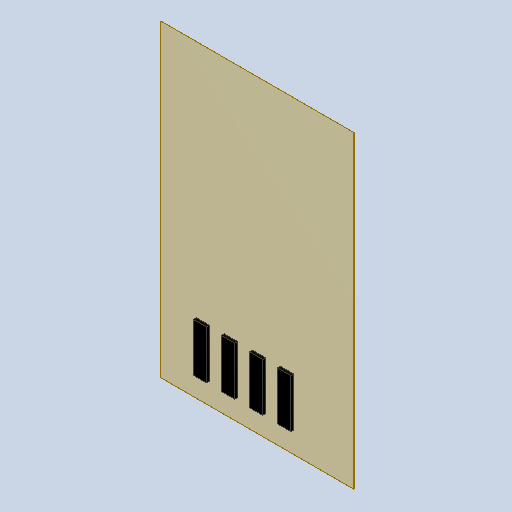
# Autodesk Inventor part: dirt
Saved by Autodesk Inventor 2025 (Build 290162010, 162A)
## iProperties
Created: 2024-06-18
Part Number: dirt
Material: 일반
Document SubType Name: Modeling
Designer: user
Density: 1 g/cm^3
Appearance: 기본값
Author: user
Autodesk Inventor part; units mm, degrees
ref_plane "YZ Plane" through (0, 0, 0) normal (1, 0, 0) x (0, 1, 0)
ref_plane "XZ Plane" through (0, 0, 0) normal (0, 1, 0) x (-1, 0, 0)
ref_plane "XY Plane" through (0, 0, 0) normal (0, 0, 1) x (1, 0, 0)
ref_plane "작업 평면1" through (2977.2317, -10029.2607, -15) normal (0, 0, 1) x (1, 0, 0)
ref_plane "작업 평면2" through (2977.2317, -10029.2607, -30) normal (0, 0, 1) x (1, 0, 0)
sketch "스케치1" plane through (2977.2317, -10029.2607, -30) normal (0, 0, 1) x (1, 0, 0)
  line L0 (5170.4623, -12069.2506) -> (3270.4623, -12069.2506)
  line L1 (3270.4623, -12069.2506) -> (3270.4623, -18969.2506)
  line L2 (3270.4623, -18969.2506) -> (5170.4623, -18969.2506)
  line L3 (5170.4623, -18969.2506) -> (5170.4623, -12069.2506)
  line L4 (1170.4623, -12069.2506) -> (-729.5377, -12069.2506)
  line L5 (-729.5377, -12069.2506) -> (-729.5377, -18969.2506)
  line L6 (-729.5377, -18969.2506) -> (1170.4623, -18969.2506)
  line L7 (1170.4623, -18969.2506) -> (1170.4623, -12069.2506)
  line L8 (-2829.5377, -12069.2506) -> (-4729.5377, -12069.2506)
  line L9 (-4729.5377, -12069.2506) -> (-4729.5377, -18969.2506)
  line L10 (-4729.5377, -18969.2506) -> (-2829.5377, -18969.2506)
  line L11 (-2829.5377, -18969.2506) -> (-2829.5377, -12069.2506)
  line L12 (-6829.5377, -12069.2506) -> (-8729.5377, -12069.2506)
  line L13 (-8729.5377, -12069.2506) -> (-8729.5377, -18969.2506)
  line L14 (-8729.5377, -18969.2506) -> (-6829.5377, -18969.2506)
  line L15 (-6829.5377, -18969.2506) -> (-6829.5377, -12069.2506)
  point P0 (-2977.2317, 10029.2607)
  dimension "d0" = 1900
  dimension "d1" = 6900
  dimension "d2" = 2100
  dimension "d3" = 1900
  dimension "d4" = 2100
  dimension "d5" = 1900
  dimension "d6" = 2100
  dimension "d7" = 1900
  constraints: 32 end point, 8 parallel, 4 horizontal, 4 perpendicular
  measures "d0" distance of L2.end L1.end
  measures "d1" distance of L1.end L0.end
  measures "d2" distance of L0.end L4.start
  measures "d3" distance of L6.end L5.end
  measures "d4" distance of L4.end L8.start
  measures "d5" distance of L10.end L9.end
  measures "d6" distance of L8.end L12.start
  measures "d7" distance of L14.end L13.end
extrude "돌출1" add sketch "스케치1" along normal blind 420
